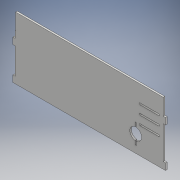
# Autodesk Inventor part: flipper-support2
Saved by Autodesk Inventor 2017 (Build 210142000, 142)
## iProperties
Created: 2017-03-05
Part Number: flipper-support2
Material: Generic
Document SubType Name: Modeling
Designer: John
Density: 1 g/cm^3
Appearance: Default
Author: John
Autodesk Inventor part; units mm, degrees
ref_plane "YZ Plane" through (0, 0, 0) normal (1, 0, 0) x (0, 1, 0)
ref_plane "XZ Plane" through (0, 0, 0) normal (0, 1, 0) x (-1, 0, 0)
ref_plane "XY Plane" through (0, 0, 0) normal (0, 0, 1) x (1, 0, 0)
sketch "Sketch1" plane through (0, 0, 0) normal (0, 1, 0) x (-1, 0, 0)
  line L0 (0, 0) -> (271, 0)
  line L1 (271, 0) -> (271, 84)
  line L2 (271, 84) -> (0, 84)
  line L3 (0, 84) -> (0, 0)
  line L4 (135.5, 84) -> (135.5, 0) construction
  line L5 (0, 84) -> (-4, 84)
  line L6 (-4, 84) -> (-4, 72)
  line L7 (-4, 72) -> (0, 72)
  line L8 (0, 72) -> (0, 84)
  line L9 (0, 0) -> (-4, 0)
  line L10 (-4, 0) -> (-4, 12)
  line L11 (-4, 12) -> (0, 12)
  line L12 (0, 12) -> (0, 0)
  line L13 (271, 84) -> (271, 0)
  line L14 (275, 72) -> (275, 60)
  line L15 (275, 60) -> (271, 60)
  line L16 (271, 60) -> (271, 84)
  line L17 (271, 0) -> (275, 0)
  line L18 (275, 0) -> (275, 12)
  line L19 (275, 12) -> (271, 12)
  line L20 (271, 12) -> (271, 0)
  arc A0 (51.367, 20.056) -> (49.367, 20.056) centre (50.367, 20.056) ccw
  arc A1 (49.367, 41.706) -> (51.367, 41.706) centre (50.367, 41.706) ccw
  line L21 (49.367, 48.706) -> (49.367, 41.706)
  line L22 (50.367, 41.706) -> (50.367, 48.706) construction
  line L23 (51.367, 41.706) -> (51.367, 48.706)
  arc A2 (51.367, 48.706) -> (49.367, 48.706) centre (50.367, 48.706) ccw
  circle A3 centre (50.367, 30.881) radius 10.825
  arc A4 (49.367, 13.056) -> (51.367, 13.056) centre (50.367, 13.056) ccw
  line L24 (49.367, 20.056) -> (49.367, 13.056)
  line L25 (50.367, 20.056) -> (50.367, 13.056) construction
  line L26 (51.367, 13.056) -> (51.367, 20.056)
  line L27 (275, 72) -> (271, 72)
  point P0 (50.367, 45.206)
  point P1 (50.367, 16.556)
  dimension "d0" = 271
  dimension "d2" = 4
  dimension "d3" = 12
  dimension "d4" = 4
  dimension "d5" = 12
  dimension "d20" = 21.65
  dimension "d21" = 7
  dimension "d22" = 2
  dimension "d23" = 7
  dimension "d24" = 2
  dimension "d56" = 50.367
  dimension "d57" = 30.881
  dimension "d58" = 48
  dimension "d59" = 12
  dimension "d60" = 12
  constraints: 60 end point, 10 point on circle, 8 parallel, 8 tangent, 5 centre point, 5 midpoint, 3 horizontal, 3 perpendicular, 2 vertical, 1 coincident
  measures "d0" distance of L2.end L1.end
  measures "d2" distance of L7.end L6.end
  measures "d3" distance of L6.end L5.end
  measures "d4" distance of L10.end L11.end
  measures "d5" distance of L9.end L10.end
  measures "d20" diameter of A3
  measures "d21" distance of L22.start L22.end
  measures "d22" diameter of A2
  measures "d23" distance of L25.start L25.end
  measures "d24" diameter of A4
  measures "d56" distance from line of L3 A3.centre
  measures "d57" distance from line of L0 point (50.367, 30.881)
  measures "d58" distance between parallel lines of L15 L19
  measures "d59" distance of L17.end L18.end
  measures "d60" distance of L14.start L14.end
extrude "Extrusion1" add sketch "Sketch1" along normal blind 3
sketch "Sketch3" plane through (0, 0, 0) normal (0, -1, 0) x (1, 0, 0)
  line L0 (4, 0) -> (-275, 0) projected
  line L1 (-270, 114) -> (0, 114)
  line L2 (0, 114) -> (0, 84)
  line L3 (0, 84) -> (-270, 84)
  line L4 (-270, 84) -> (-270, 114)
  line L5 (-275, 84) -> (4, 84) projected
  point P0 (0, 0)
  point P1 (-275, 72)
  point P2 (4, 84)
  dimension "d28" = 30
  constraints: 8 end point, 2 parallel, 1 collinear, 1 horizontal, 1 perpendicular
  measures "d28" distance of L1.end L2.end
extrude "Extrusion2" add sketch "Sketch3" against normal blind 3
sketch "Sketch2" plane through (0, 0, 0) normal (0, -1, 0) x (1, 0, 0)
  circle A0 centre (-25.367, 65.881) radius 1.5 construction
  arc A1 (-49.3681, 20.1022) -> (-49.3681, 41.6598) centre (-50.367, 30.881) ccw construction
  line L0 (-8.367, 65.881) -> (-42.367, 65.881) construction
  line L1 (-8.367, 67.381) -> (-42.367, 67.381)
  line L2 (-42.367, 64.381) -> (-8.367, 64.381)
  arc A2 (-8.367, 64.381) -> (-8.367, 67.381) centre (-8.367, 65.881) ccw
  arc A3 (-42.367, 67.381) -> (-42.367, 64.381) centre (-42.367, 65.881) ccw
  line L3 (-8.367, 82.381) -> (-42.367, 82.381) construction
  line L4 (-8.367, 83.881) -> (-42.367, 83.881)
  line L5 (-42.367, 80.881) -> (-8.367, 80.881)
  arc A4 (-8.367, 80.881) -> (-8.367, 83.881) centre (-8.367, 82.381) ccw
  arc A5 (-42.367, 83.881) -> (-42.367, 80.881) centre (-42.367, 82.381) ccw
  line L6 (-8.367, 49.381) -> (-42.367, 49.381) construction
  line L7 (-8.367, 50.881) -> (-42.367, 50.881)
  line L8 (-42.367, 47.881) -> (-8.367, 47.881)
  arc A6 (-8.367, 47.881) -> (-8.367, 50.881) centre (-8.367, 49.381) ccw
  arc A7 (-42.367, 50.881) -> (-42.367, 47.881) centre (-42.367, 49.381) ccw
  line L9 (-42.367, 65.881) -> (-42.367, 49.381) construction
  line L10 (-42.367, 82.381) -> (-42.367, 65.881) construction
  point P0 (0, 0)
  point P1 (-25.367, 82.381)
  point P2 (-25.367, 49.381)
  dimension "d41" = 3
  dimension "d43" = 25
  dimension "d44" = 35
  dimension "d45" = 17
  dimension "d46" = 3
  dimension "d47" = 17
  dimension "d48" = 3
  dimension "d52" = 17
  dimension "d53" = 3
  dimension "d54" = 16.5
  dimension "d55" = 16.5
  constraints: 28 end point, 12 point on circle, 12 tangent, 7 centre point, 3 horizontal, 3 midpoint, 3 parallel, 2 vertical
  measures "d41" diameter of A0
  measures "d43" horizontal distance of A1.centre A0.centre
  measures "d44" vertical distance of A1.centre A0.centre
  measures "d45" distance of A0.centre L0.end
  measures "d46" diameter of A3
  measures "d47" distance of point (-25.367, 82.381) L3.end
  measures "d48" diameter of A5
  measures "d52" distance of point (-25.367, 49.381) L6.end
  measures "d53" diameter of A7
  measures "d54" distance between parallel lines of L0 L6
  measures "d55" distance between parallel lines of L3 L0
extrude "Extrusion3" cut sketch "Sketch2" against normal blind 3
equation "\"d4\" = d2"
equation "\"d41\" = d40"
equation "\"d45\" = d52"
equation "\"d47\" = d52"
equation "\"d40\" = 3"
body "Solid1"
